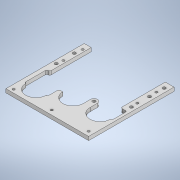
# Autodesk Inventor part: Bottle layout
Saved by Autodesk Inventor 2021 (Build 250183000, 183)
## iProperties
Created: 2020-07-28
Part Number: Bottle layout
Material: Generic
Document SubType Name: Modeling
Designer: jgray
Density: 1 g/cm^3
Appearance: Default
Author: jgray
Autodesk Inventor part; units mm, degrees
ref_plane "YZ Plane" through (0, 0, 0) normal (1, 0, 0) x (0, 1, 0)
ref_plane "XZ Plane" through (0, 0, 0) normal (0, 1, 0) x (-1, 0, 0)
ref_plane "XY Plane" through (0, 0, 0) normal (0, 0, 1) x (1, 0, 0)
sketch "Sketch1" plane through (0, 0, 0) normal (0, 1, 0) x (-1, 0, 0)
  line L0 (-56.25, 58.25) -> (56.25, 58.25)
  line L1 (56.25, 58.25) -> (56.25, -58.25)
  line L2 (56.25, -58.25) -> (-56.25, -58.25)
  line L3 (-56.25, -58.25) -> (-56.25, 58.25)
  line L4 (-56.25, 58.25) -> (56.25, -58.25) construction
  line L5 (56.25, 58.25) -> (-56.25, -58.25) construction
  point P0 (0, 0)
  dimension "d0" = 112.5
  dimension "d1" = 116.5
  constraints: 12 end point, 2 midpoint, 2 parallel, 1 horizontal, 1 perpendicular
  measures "d0" distance of L1.end L2.end
  measures "d1" distance of L0.end L1.end
extrude "Extrusion1" add sketch "Sketch1" along normal blind 5
sketch "Sketch2" plane through (0, 5, 0) normal (0, 1, 0) x (1, 0, 0)
  circle A0 centre (18.5, 28) radius 23.85
  circle A1 centre (37, -23.25) radius 13.85
  circle A2 centre (-35, -38.75) radius 13.85
  circle A3 centre (-30.9, 25.8) radius 13.85
  circle A4 centre (0, -23.25) radius 13.85
  line L0 (56.25, 58.25) -> (-56.25, 58.25)
  line L1 (-56.25, -58.25) -> (56.25, -58.25)
  line L2 (0, -105.929917) -> (0, 123.208568) construction
  line L3 (-76.477668, -38.75) -> (-5.35, -38.75) construction
  line L4 (-123.544744, -23.25) -> (82.557161, -23.25) construction
  line L5 (56.25, -58.25) -> (56.25, 58.25) construction
  point P0 (0, 0)
  dimension "d4" = 47.7
  dimension "d5" = 27.7
  dimension "d6" = 27.7
  dimension "d7" = 27.7
  dimension "d8" = 27.7
  dimension "d9" = 116.5
  dimension "d10" = 112.5
  dimension "d13" = 37
  dimension "d14" = 18.5
  dimension "d15" = 30.9
  dimension "d18" = 19.5
  dimension "d19" = 35
  dimension "d20" = 35
  dimension "d157" = 25.8
  dimension "d158" = 28
  constraints: 6 end point, 5 centre point, 5 point on line, 1 horizontal, 1 perpendicular, 1 vertical
  measures "d4" diameter of A0
  measures "d5" diameter of A1
  measures "d6" diameter of A2
  measures "d7" diameter of A3
  measures "d8" diameter of A4
  measures "d9" distance between parallel lines of L0 L1
  measures "d10" distance of L1.start L1.end
  measures "d13" distance of A4.centre A1.centre
  measures "d14" distance from line of A0.centre L2
  measures "d15" distance from line of A3.centre L2
  measures "d18" distance between parallel lines of L1 L3
  measures "d19" distance between parallel lines of L1 L4
  measures "d20" horizontal distance of A2.centre A4.centre
  measures "d157" vertical distance of point (0, 0) A3.centre
  measures "d158" vertical distance of point (0, 0) A0.centre
extrude "Extrusion2" cut sketch "Sketch2" against normal blind 5
sketch "Sketch3" plane through (0, 5, 0) normal (0, 1, 0) x (1, 0, 0)
  line L0 (-56.266739, 58.25) -> (-56.266739, -58.25) construction
  circle A0 centre (0, -23.25) radius 13.85 construction
  circle A1 centre (37, -23.25) radius 13.85 construction
  circle A2 centre (-30.916739, 25.8) radius 13.85 construction
  line L1 (56.25, 58.25) -> (-56.266739, 58.25) construction
  line L2 (-17.15, -23.25) -> (-13.85, -23.25) construction
  line L3 (-46.75, -8.182153) -> (-46.85, -8.182153)
  line L4 (-13.85, -23.25) -> (-17.15, -23.25)
  line L5 (56.25, -58.25) -> (56.25, 58.25)
  line L6 (-46.85, -8.182153) -> (-46.766739, -8.182153)
  arc A3 (-13.85, -23.25) -> (13.85, -23.25) centre (0, -23.25) ccw
  arc A4 (23.15, -23.25) -> (50.85, -23.25) centre (37, -23.25) ccw
  line L7 (-44.75, 58.25) -> (42.35, 58.25)
  line L8 (-48.866739, -40.25) -> (-48.866739, -40.25)
  line L9 (-50.866739, -38.75) -> (-50.866739, -10.198892)
  line L10 (-48.85, -8.182153) -> (-48.766739, -8.182153)
  arc A5 (-48.85, -8.182153) -> (-50.866739, -10.198892) centre (-48.85, -10.198892) ccw
  line L11 (50.85, -23.25) -> (50.85, -23.25)
  line L12 (52.85, -21.25) -> (52.85, -4.75)
  line L13 (50.85, -2.75) -> (46.35, -2.75)
  arc A6 (50.85, -23.25) -> (52.85, -21.25) centre (50.85, -21.25) ccw
  arc A7 (52.85, -4.75) -> (50.85, -2.75) centre (50.85, -4.75) ccw
  line L14 (-44.751621, 25.8) -> (-44.751621, 25.8)
  line L15 (-46.766739, 28.033923) -> (-46.766739, 58.25)
  line L16 (-44.75, 58.25) -> (-46.766739, 58.25)
  line L17 (-17.073359, 26.228188) -> (-17.056621, 26.228188)
  line L18 (-15.066739, 27.8) -> (-15.066739, 58.25)
  line L19 (-5.349992, 27.98) -> (-5.349991, 27.98)
  line L20 (-7.35, 29.979635) -> (-7.35, 58.25)
  line L21 (42.349991, 27.98) -> (42.35, 27.98)
  line L22 (44.35, 58.25) -> (42.35, 58.25)
  circle A8 centre (0, -23.25) radius 13.85
  circle A9 centre (37, -23.25) radius 13.85
  line L23 (44.35, 58.25) -> (44.35, -0.75)
  line L24 (42.35, 27.98) -> (44.35, 27.98)
  line L25 (-5.349991, 27.98) -> (-5.349999, 27.98)
  line L26 (-7.35, 29.98) -> (-7.35, 29.979635)
  line L27 (-17.056621, 26.228188) -> (-17.056621, 26.228188)
  line L28 (-46.766739, 28.033923) -> (-46.766739, -6.182153)
  arc A10 (-48.766739, -8.182153) -> (-46.766739, -6.182153) centre (-48.766739, -6.182153) ccw
  line L29 (-44.766739, 25.8) -> (-46.766739, 25.8)
  line L30 (-21.15, -40.25) -> (-21.15, -40.25)
  line L31 (-19.166739, -36.75) -> (-19.166739, -25.266739)
  arc A11 (-17.15, -23.25) -> (-19.166739, -25.266739) centre (-17.15, -25.266739) ccw
  line L32 (-17.066739, 25.8) -> (-17.066739, 25.8)
  arc A12 (-17.066739, 25.8) -> (-15.066739, 27.8) centre (-17.066739, 27.8) ccw
  line L33 (-56.266739, -58.25) -> (56.25, -58.25)
  line L34 (56.25, -58.25) -> (56.25, 58.25)
  line L35 (56.25, 58.25) -> (-56.266739, 58.25)
  line L36 (-56.266739, 58.25) -> (-56.266739, -58.25)
  circle A13 centre (-30.916739, 25.8) radius 13.85
  circle A14 centre (-30.916739, 25.8) radius 13.85
  line L37 (13.85, -23.25) -> (13.85, -13.25)
  circle A15 centre (0, -23.25) radius 13.85
  line L38 (23.15, -23.25) -> (23.15, -13.25)
  circle A16 centre (37, -23.25) radius 13.85
  arc A17 (23.15, -13.25) -> (13.85, -13.25) centre (18.5, -13.25) ccw
  circle A18 centre (18.5, 28) radius 23.85
  circle A19 centre (18.5, 28) radius 23.85
  line L39 (56.25, 58.25) -> (-56.266739, 58.25)
  circle A20 centre (-35, -38.75) radius 13.85
  circle A21 centre (-35, -38.75) radius 13.85
  arc A22 (44.35, -0.75) -> (46.35, -2.75) centre (46.35, -0.75) ccw
  line L40 (-5.349999, 27.98) -> (-5.35, 27.98)
  arc A23 (-7.35, 29.98) -> (-5.35, 27.98) centre (-5.35, 29.98) ccw
  line L41 (-56.266739, 58.25) -> (-56.266739, -58.25) construction
  circle A24 centre (-0.016739, -23.25) radius 13.85 construction
  circle A25 centre (36.983261, -23.25) radius 13.85 construction
  circle A26 centre (-30.916739, 25.8) radius 13.85 construction
  line L42 (56.233261, 58.25) -> (-56.266739, 58.25) construction
  line L43 (-17.166739, -23.25) -> (-13.866739, -23.25) construction
  line L44 (-46.75, -8.182153) -> (-46.85, -8.182153)
  line L45 (-13.866739, -23.25) -> (-17.166739, -23.25)
  line L46 (56.233261, -58.25) -> (56.233261, 58.25)
  line L47 (-46.866739, -8.182153) -> (-46.766739, -8.182153)
  arc A27 (-13.866739, -23.25) -> (13.833261, -23.25) centre (-0.016739, -23.25) ccw
  arc A28 (23.133261, -23.25) -> (50.833261, -23.25) centre (36.983261, -23.25) ccw
  line L48 (-44.766739, 58.25) -> (42.333261, 58.25)
  line L49 (-48.85, -40.25) -> (-48.85, -40.25)
  line L50 (-50.866739, -36.75) -> (-50.866739, -10.182153)
  line L51 (-48.866739, -8.182153) -> (-48.766739, -8.182153)
  arc A29 (-48.866739, -8.182153) -> (-50.866739, -10.182153) centre (-48.866739, -10.182153) ccw
  line L52 (50.833261, -23.25) -> (50.833261, -23.25)
  line L53 (52.833261, -21.25) -> (52.833261, -4.75)
  line L54 (50.833261, -2.75) -> (46.333261, -2.75)
  arc A30 (50.833261, -23.25) -> (52.833261, -21.25) centre (50.833261, -21.25) ccw
  arc A31 (52.833261, -4.75) -> (50.833261, -2.75) centre (50.833261, -4.75) ccw
  line L55 (-44.76836, 25.8) -> (-44.76836, 25.8)
  line L56 (-46.766739, 28.033923) -> (-46.766739, 58.25)
  line L57 (-44.766739, 58.25) -> (-46.766739, 58.25)
  line L58 (-17.073359, 26.228188) -> (-17.073359, 26.228188)
  line L59 (-15.066739, 27.8) -> (-15.066739, 58.25)
  line L60 (-5.36673, 27.98) -> (-5.366729, 27.98)
  line L61 (-7.366739, 29.979635) -> (-7.366739, 58.25)
  line L62 (42.333252, 27.98) -> (42.333261, 27.98)
  line L63 (44.333261, 58.25) -> (42.333261, 58.25)
  circle A32 centre (-0.016739, -23.25) radius 13.85
  circle A33 centre (36.983261, -23.25) radius 13.85
  line L64 (44.333261, 58.25) -> (44.333261, -0.75)
  line L65 (42.333261, 27.98) -> (44.333261, 27.98)
  line L66 (-5.366729, 27.98) -> (-5.366738, 27.98)
  line L67 (-7.366739, 29.98) -> (-7.366739, 29.979635)
  line L68 (-17.073359, 26.228188) -> (-17.073359, 26.228188)
  line L69 (-15.066739, 28.002891) -> (-15.066739, 28.002891)
  line L70 (-46.766739, 28.033923) -> (-46.766739, -6.182153)
  arc A34 (-48.766739, -8.182153) -> (-46.766739, -6.182153) centre (-48.766739, -6.182153) ccw
  line L71 (-44.766739, 25.8) -> (-46.766739, 25.8)
  line L72 (-21.15, -40.25) -> (-21.15, -40.25)
  line L73 (-19.166739, -38.25) -> (-19.166739, -25.25)
  arc A35 (-17.166739, -23.25) -> (-19.166739, -25.25) centre (-17.166739, -25.25) ccw
  line L74 (-17.066739, 25.8) -> (-17.066739, 25.8)
  arc A36 (-17.066739, 25.8) -> (-15.066739, 27.8) centre (-17.066739, 27.8) ccw
  line L75 (-56.266739, -58.25) -> (56.233261, -58.25)
  line L76 (56.233261, -58.25) -> (56.233261, 58.25)
  line L77 (56.233261, 58.25) -> (-56.266739, 58.25)
  line L78 (-56.266739, 58.25) -> (-56.266739, -58.25)
  circle A37 centre (-30.9, 25.8) radius 13.833261
  circle A38 centre (-30.9, 25.8) radius 13.833261
  line L79 (13.833261, -23.25) -> (13.833261, -13.25)
  circle A39 centre (-0.016739, -23.25) radius 13.85
  line L80 (23.133261, -23.25) -> (23.133261, -13.25)
  circle A40 centre (36.983261, -23.25) radius 13.85
  arc A41 (23.133261, -13.25) -> (13.833261, -13.25) centre (18.483261, -13.25) ccw
  circle A42 centre (18.483261, 28) radius 23.85
  circle A43 centre (18.483261, 28) radius 23.85
  line L81 (56.233261, 58.25) -> (-56.266739, 58.25)
  circle A44 centre (-35, -38.75) radius 13.85
  arc A45 (44.333261, -0.75) -> (46.333261, -2.75) centre (46.333261, -0.75) ccw
  line L82 (-5.366738, 27.98) -> (-5.366739, 27.98)
  arc A46 (-7.366739, 29.98) -> (-5.366739, 27.98) centre (-5.366739, 29.98) ccw
  circle A47 centre (18.5, 28) radius 23.85
  circle A48 centre (37, -23.25) radius 13.85
  circle A49 centre (-30.9, 25.8) radius 13.85
  circle A50 centre (0, -23.25) radius 13.85
  circle A51 centre (-35, -38.75) radius 13.85
  line L83 (56.25, 58.25) -> (-56.25, 58.25)
  line L84 (-56.25, 58.25) -> (-56.25, -58.25)
  line L85 (-56.25, -58.25) -> (56.25, -58.25)
  line L86 (56.25, -58.25) -> (56.25, 58.25)
  line L87 (-48.866739, -38.75) -> (-21.166739, -38.75)
  line L88 (-56.25, 58.25) -> (-56.25, -58.25)
  line L89 (-56.25, -58.25) -> (56.25, -58.25)
  line L90 (56.25, -58.25) -> (56.25, 58.25)
  line L91 (56.25, 58.25) -> (-56.25, 58.25)
  circle A52 centre (-30.9, 25.8) radius 13.85
  circle A53 centre (18.5, 28) radius 23.85
  circle A54 centre (-35, -38.75) radius 13.85
  circle A55 centre (0, -23.25) radius 13.85
  circle A56 centre (37, -23.25) radius 13.85
  arc A57 (-21.166739, -38.75) -> (-19.166739, -36.75) centre (-21.166739, -36.75) ccw
  arc A58 (-50.866739, -36.75) -> (-48.866739, -38.75) centre (-48.866739, -36.75) ccw
  point P0 (18.5, 27.979635)
  point P1 (-30.9, 25.819804)
  point P2 (-0.016739, 0)
  point P3 (0, 0)
  point P4 (44.35, -2.75)
  point P5 (52.85, -23.25)
  point P6 (-15.066739, 28.002891)
  point P7 (-15.066739, 28.002891)
  point P8 (50.85, -23.25)
  point P9 (-19.166739, -38.25)
  point P10 (50.85, -23.25)
  point P11 (-46.75, 58.25)
  point P12 (-46.75, 58.25)
  point P13 (50.85, -23.25)
  point P14 (-44.75, 25.8)
  point P15 (-17.05, 25.8)
  point P16 (-7.35, 27.98)
  point P17 (-7.35, 29.98)
  point P18 (-21.15, -40.25)
  point P19 (-0.016739, 0)
  point P20 (-0.016739, 0)
  point P21 (44.333261, -2.75)
  point P22 (52.833261, -23.25)
  point P23 (50.85, -23.25)
  point P24 (50.85, -23.25)
  point P25 (-46.75, 58.25)
  point P26 (-46.75, 58.25)
  point P27 (50.85, -23.25)
  point P28 (-44.75, 25.8)
  point P29 (-17.05, 25.8)
  point P30 (-7.366739, 27.98)
  point P31 (-7.35, 29.98)
  point P32 (-21.15, -40.25)
  point P33 (42.35, 28)
  point P34 (-5.349998, 27.989818)
  point P35 (13.85, -23.25)
  point P36 (50.85, -23.25)
  point P37 (-30.908369, 11.950003)
  point P38 (-30.908369, 39.649997)
  point P39 (-19.166739, -38.75)
  point P40 (50.85, -23.24993)
  point P41 (-48.85, -38.75)
  point P42 (-21.15, -38.74993)
  dimension "d95" = 27.7
  dimension "d96" = 27.7
  dimension "d134" = 27.7
  dimension "d135" = 27.7
  dimension "d81" = 2
  dimension "d82" = 2
  dimension "d83" = 2
  dimension "d84" = 2
  dimension "d86" = 2
  dimension "d87" = 2
  dimension "d88" = 27.7
  dimension "d89" = 10
  dimension "d90" = 10
  dimension "d91" = 25.8
  dimension "d92" = 23.25
  dimension "d93" = 23.25
  dimension "d94" = 37
  dimension "d97" = 19.15
  dimension "d98" = 50.85
  dimension "d99" = 46.75
  dimension "d100" = 2.017
  dimension "d101" = 6.18215
  dimension "d102" = 31.7
  dimension "d103" = 51.7
  dimension "d104" = 30.9
  dimension "d105" = 3.4
  dimension "d106" = 11.9
  dimension "d107" = 61
  dimension "d108" = 47.7
  dimension "d109" = 28
  dimension "d110" = 18.5
  dimension "d111" = 30.27
  dimension "d112" = 27.7
  dimension "d113" = 2
  dimension "d114" = 30.27
  dimension "d115" = 2
  dimension "d116" = 112.51674
  dimension "d117" = 116.5
  dimension "d120" = 2
  dimension "d121" = 2
  dimension "d122" = 2
  dimension "d123" = 2
  dimension "d125" = 2
  dimension "d126" = 2
  dimension "d127" = 27.7
  dimension "d128" = 10
  dimension "d129" = 10
  dimension "d130" = 25.8
  dimension "d131" = 23.25
  dimension "d132" = 23.25
  dimension "d133" = 37
  dimension "d136" = 19.15
  dimension "d137" = 50.85
  dimension "d138" = 46.75
  dimension "d139" = 2
  dimension "d140" = 6.18215
  dimension "d141" = 31.7
  dimension "d142" = 51.7
  dimension "d143" = 30.88326
  dimension "d144" = 3.4
  dimension "d145" = 11.9
  dimension "d146" = 61
  dimension "d147" = 47.7
  dimension "d148" = 28
  dimension "d149" = 18.5
  dimension "d150" = 30.27
  dimension "d152" = 2
  dimension "d153" = 30.27
  constraints: 164 end point, 67 point on circle, 48 tangent, 45 point on line, 40 centre point, 30 perpendicular, 19 horizontal, 11 coincident, 10 vertical, 6 parallel, 4 collinear, 4 horizontal alignment, 3 equal radius, 2 concentric, 2 line through centre, 2 midpoint, 32 other
  measures "d81" distance of L11.start point (52.85, -23.25)
  measures "d82" radius of A6
  measures "d83" distance from line of L21.end L23
  measures "d84" radius of A10
  measures "d86" distance from line of L18 L32.start
  measures "d87" radius of A12
  measures "d88" diameter of A2
  measures "d89" distance of L37.start L37.end
  measures "d90" distance of L38.start L38.end
  measures "d91" vertical distance of point (-0.017, 0) A2.centre
  measures "d92" vertical distance of point (-0.017, 0) A1.centre
  measures "d93" distance of point (0, 0) A0.centre
  measures "d94" horizontal distance of A1.centre point (0, 0)
  measures "d97" distance from line of L31 point (-0.017, 0)
  measures "d98" distance from line of L9 point (-0.017, 0)
  measures "d99" distance from line of L28 point (-0.017, 0)
  measures "d101" vertical distance of point (-0.017, 0) A10.centre
  measures "d102" distance between parallel lines of L18 L15
  measures "d103" distance between parallel lines of L23 L20
  measures "d104" horizontal distance of point (-0.017, 0) point (-30.917, 25.8)
  measures "d105" distance between parallel lines of L5 L12
  measures "d106" distance between parallel lines of L5 L23
  measures "d107" distance between parallel lines of L1 L13
  measures "d108" diameter of A18
  measures "d109" vertical distance of point (0, 0) A19.centre
  measures "d110" horizontal distance of A19.centre point (0, 0)
  measures "d111" distance between parallel lines of L7 L24
  measures "d112" diameter of A20
  measures "d113" radius of A22
  measures "d114" distance of L20.end point (-7.35, 27.98)
  measures "d115" radius of A23
  measures "d116" distance between parallel lines of L34 L0
  measures "d117" distance between parallel lines of L35 L33
  measures "d120" distance of L52.start point (52.833, -23.25)
  measures "d121" radius of A30
  measures "d122" distance from line of L62.end L64
  measures "d123" radius of A34
  measures "d125" distance from line of L59 L74.start
  measures "d126" radius of A36
  measures "d127" diameter of A26
  measures "d128" distance of L79.start L79.end
  measures "d129" distance of L80.start L80.end
  measures "d130" vertical distance of point (-0.017, 0) A26.centre
  measures "d131" vertical distance of point (-0.017, 0) A25.centre
  measures "d132" distance of point (-0.017, 0) A24.centre
  measures "d133" horizontal distance of A25.centre point (-0.017, 0)
  measures "d136" distance from line of L73 point (-0.017, 0)
  measures "d137" distance from line of L50 point (-0.017, 0)
  measures "d138" distance from line of L70 point (-0.017, 0)
  measures "d139" radius of A29
  measures "d140" vertical distance of point (-0.017, 0) A34.centre
  measures "d141" distance between parallel lines of L59 L56
  measures "d142" distance between parallel lines of L64 L61
  measures "d143" horizontal distance of point (-0.017, 0) A37.centre
  measures "d144" distance between parallel lines of L46 L53
  measures "d145" distance between parallel lines of L46 L64
  measures "d146" distance between parallel lines of L42 L54
  measures "d147" diameter of A42
  measures "d148" vertical distance of point (-0.017, 0) A43.centre
  measures "d149" horizontal distance of A43.centre point (-0.017, 0)
  measures "d150" distance between parallel lines of L48 L65
  measures "d152" radius of A45
  measures "d153" distance of L61.end point (-7.367, 27.98)
sketch "Sketch3 outline for Extrusion3" plane through (0, 5, 0) normal (0, 1, 0) x (1, 0, 0)
  arc A0 (23.15, -23.25) -> (50.85, -23.25) centre (37, -23.25) cw
  line L0 (23.15, -13.25) -> (23.15, -23.25)
  arc A1 (50.85, -23.25) -> (52.85, -21.25) centre (50.85, -21.25) ccw
  arc A2 (13.85, -13.25) -> (23.15, -13.25) centre (18.5, -13.25) cw
  line L1 (52.85, -21.25) -> (52.85, -4.75)
  line L2 (13.85, -23.25) -> (13.85, -13.25)
  arc A3 (52.85, -4.75) -> (50.85, -2.75) centre (50.85, -4.75) ccw
  arc A4 (-13.85, -23.25) -> (13.85, -23.25) centre (0, -23.25) cw
  line L3 (50.85, -2.75) -> (50.833261, -2.75)
  line L4 (-17.15, -23.25) -> (-13.85, -23.25)
  line L5 (50.833261, -2.75) -> (46.35, -2.75)
  arc A5 (-19.166739, -25.266739) -> (-17.15, -23.25) centre (-17.15, -25.266739) cw
  arc A6 (46.35, -2.75) -> (44.35, -0.75) centre (46.35, -0.75) cw
  line L6 (-19.166739, -36.75) -> (-19.166739, -25.266739)
  line L7 (44.35, -0.75) -> (44.35, 58.25)
  arc A7 (-21.15, -38.74993) -> (-19.166739, -36.75) centre (-21.166739, -36.75) ccw
  line L8 (44.35, 58.25) -> (44.333261, 58.25)
  arc A8 (-48.85, -38.75) -> (-21.15, -38.74993) centre (-35, -38.75) cw
  line L9 (44.333261, 58.25) -> (42.333261, 58.25)
  line L10 (-48.866739, -38.75) -> (-48.85, -38.75)
  line L11 (42.333261, 58.25) -> (-44.766739, 58.25)
  arc A9 (-50.866739, -36.75) -> (-48.866739, -38.75) centre (-48.866739, -36.75) ccw
  line L12 (-44.766739, 58.25) -> (-46.766739, 58.25)
  line L13 (-50.866739, -10.198892) -> (-50.866739, -36.75)
  line L14 (-46.766739, 58.25) -> (-46.766739, 28.033923)
  arc A10 (-48.85, -8.182153) -> (-50.866739, -10.198892) centre (-48.85, -10.198892) ccw
  line L15 (-46.766739, 28.033923) -> (-46.766739, -6.182153)
  line L16 (-48.766739, -8.182153) -> (-48.85, -8.182153)
  arc A11 (-46.766739, -6.182153) -> (-48.766739, -8.182153) centre (-48.766739, -6.182153) cw
  arc A12 (-30.908369, 39.649997) -> (-30.908369, 11.950003) centre (-30.916739, 25.8) cw
  arc A13 (-30.908369, 11.950003) -> (-30.908369, 39.649997) centre (-30.9, 25.8) cw
  arc A14 (-5.349998, 27.989818) -> (42.35, 28) centre (18.5, 28) cw
  arc A15 (42.35, 28) -> (-5.349998, 27.989818) centre (18.5, 28) cw
extrude "Extrusion3" cut sketch "Sketch3 outline for Extrusion3" against normal blind 5
sketch "Sketch4" plane through (0, 5, 0) normal (0, 1, 0) x (1, 0, 0)
  line L0 (-56.25, 58.25) -> (-56.25, -58.25)
  line L1 (56.25, -58.25) -> (56.25, 58.25)
  line L2 (-51.55, 5.4) -> (-51.55, 71.994123) construction
  line L3 (50.75, 5.4) -> (50.75, 69.456542) construction
  line L4 (-73.721988, 50) -> (66.546719, 50) construction
  line L5 (66.546719, 30) -> (-76.077923, 30) construction
  line L6 (18.5, -1.340599) -> (18.5, -39.445861) construction
  line L7 (6.353115, -13.25) -> (33.621097, -13.25) construction
  point P0 (0, 0)
  point P1 (-51.55, 30)
  point P2 (50.75, 50)
  point P3 (50.75, 30)
  point P4 (18.5, -13.25)
  dimension "d48" = 4.7
  dimension "d49" = 5.5
  dimension "d58" = 30
  dimension "d59" = 50
  dimension "d72" = 5.4
  dimension "d73" = 5.4
  constraints: 12 end point, 8 point on line, 3 horizontal, 3 vertical
  measures "d48" distance from line of L0 L2.start
  measures "d49" distance from line of L1 L3.start
  measures "d58" distance from line of point (0, 0) L5
  measures "d59" distance from line of point (0, 0) L4
  measures "d72" vertical distance of point (0, 0) L3.start
  measures "d73" vertical distance of point (0, 0) L2.start
hole "Hole1" at (-51.55, 5, -5.4) at (50.75, 5, -5.4) at (-51.55, 5, -30) at (50.75, 5, -50) at (50.75, 5, -30) at (18.5, 5, 13.25) direction (0, -1, 0) diameter 4.2 end through all
sketch "Sketch5" plane through (0, 5, 0) normal (0, 1, 0) x (1, 0, 0)
  line L0 (-50.25, 75.94977) -> (-50.25, -88.006053) construction
  line L1 (-63.914485, -52.25) -> (79.409686, -52.25) construction
  line L2 (50.25, 66.292399) -> (50.25, -77.90971) construction
  line L3 (-56.25, 58.25) -> (-56.25, -58.25) construction
  line L4 (-56.25, -58.25) -> (56.25, -58.25) construction
  line L5 (56.25, -58.25) -> (56.25, 58.25) construction
  line L6 (-71.815971, 40) -> (84.238372, 40) construction
  line L7 (-70.718543, 14) -> (79.409686, 14) construction
  point P0 (0, 0)
  point P1 (-50.25, 40)
  point P2 (-50.25, 14)
  point P3 (-50.25, -53.75)
  point P4 (50.25, -52.25)
  point P5 (0, -52.25)
  point P6 (50.25, 14)
  point P7 (50.25, 40)
  dimension "d1" = 116.5
  dimension "d60" = 6
  dimension "d61" = 6
  dimension "d62" = 6
  dimension "d63" = 14
  dimension "d64" = 40
  dimension "d162" = 58.25
  dimension "d163" = 4.5
  constraints: 12 point on line, 10 end point, 3 horizontal, 2 vertical
  measures "d60" distance between parallel lines of L3 L0
  measures "d61" distance between parallel lines of L4 L1
  measures "d62" distance between parallel lines of L5 L2
  measures "d63" distance from line of point (0, 0) L7
  measures "d64" distance from line of point (0, 0) L6
  measures "d162" distance from line of point (0, 0) L4
  measures "d163" distance from line of point (-50.25, -53.75) L4
hole "Hole2" at (-50.25, 5, -40) at (-50.25, 5, -14) at (-50.25, 5, 53.75) at (50.25, 5, 52.25) at (0, 5, 52.25) at (50.25, 5, -14) at (50.25, 5, -40) direction (0, -1, 0) diameter 3.2 end through all
sketch "Sketch6" plane through (0, 5, 0) normal (0, 1, 0) x (1, 0, 0)
  line L0 (56.25, 58.25) -> (-56.25, 58.25)
  line L1 (-56.25, 58.25) -> (-46.766739, 58.25)
  line L2 (-46.766739, 58.25) -> (-46.766739, 48.25)
  line L3 (-46.766739, 48.25) -> (-56.25, 48.25)
  line L4 (-56.25, 48.25) -> (-56.25, 58.25)
  line L5 (-56.25, 58.25) -> (-56.25, -58.25)
  line L6 (-46.766739, -6.182153) -> (-46.766739, 58.25)
  point P0 (0, 0)
  point P1 (-46.75, 58.25)
  dimension "d159" = 10
  constraints: 8 end point, 2 parallel, 1 collinear, 1 horizontal, 1 perpendicular, 1 point on line
  measures "d159" distance of L1.end L2.end
extrude "Extrusion4" cut sketch "Sketch6" against normal blind 10
sketch "Sketch7" plane through (56.25, 0, -58.25) normal (0, 0, -1) x (-1, 0, 0)
  line L0 (0, 0) -> (0, 5) projected
  line L1 (11.9, 5) -> (11.9, 0) projected
  line L2 (0, 5) -> (11.9, 5)
  line L3 (11.9, 5) -> (11.9, 0)
  line L4 (11.9, 0) -> (0, 0)
  line L5 (0, 0) -> (0, 5)
  point P0 (56.25, 0)
  constraints: 8 end point, 2 parallel, 1 horizontal, 1 perpendicular
extrude "Extrusion5" cut sketch "Sketch7" against normal blind 0.3
body "Solid1"
